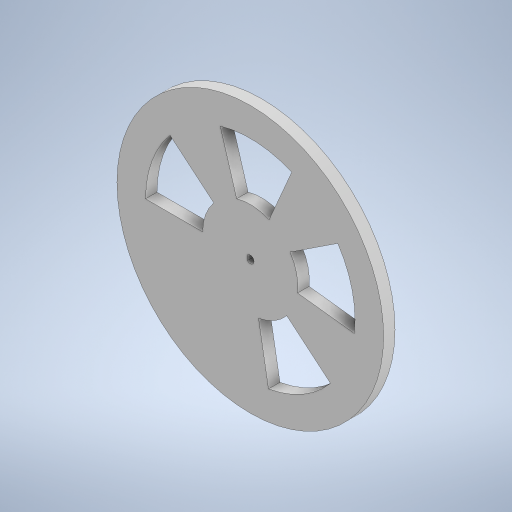
# Autodesk Inventor part: back_cir_hold2
Saved by Autodesk Inventor 2024 (Build 280153000, 153)
## iProperties
Created: 2024-03-23
Part Number: back_cir_hold2
Material: Generic
Document SubType Name: Modeling
Designer: op04o
Density: 1 g/cm^3
Appearance: Default
Author: op04o
Autodesk Inventor part; units mm, degrees
ref_plane "YZ Plane" through (0, 0, 0) normal (1, 0, 0) x (0, 1, 0)
ref_plane "XZ Plane" through (0, 0, 0) normal (0, 1, 0) x (-1, 0, 0)
ref_plane "XY Plane" through (0, 0, 0) normal (0, 0, 1) x (1, 0, 0)
sketch "Sketch1" plane through (0, 0, 0) normal (0, 0, 1) x (1, 0, 0)
  arc A0 (-1.5, -1.3229) -> (-1.5, 1.3229) centre (0, 0) ccw
  line L0 (-1.5, 1.3229) -> (-1.5, -1.3229)
  circle A1 centre (0, 0) radius 70
  dimension "d0" = 4
  dimension "d1" = 1.5
  dimension "d2" = 140
  constraints: 6 coincident, 2 centre point, 2 end point, 2 point on circle, 1 vertical
  measures "d0" diameter of A0
  measures "d1" distance from line of point (0, 0) L0
  measures "d2" diameter of A1
extrude "Extrusion1" add sketch "Sketch1" along normal blind 6
sketch "Sketch2" plane through (0, 0, 0) normal (0, 0, -1) x (-1, 0, 0)
  circle A0 centre (0, 0) radius 70 construction
  arc A1 (1.5, 1.3229) -> (1.5, -1.3229) centre (0, 0) ccw construction
  circle A2 centre (0, 0) radius 70
  line L0 (1.5, -1.3229) -> (1.5, 1.3229) construction
  arc A3 (1.5, 1.3229) -> (1.5, -1.3229) centre (0, 0) ccw construction
  line L1 (0, 0) -> (-1.5321, 1.2856)
  arc A4 (55, 0) -> (42.1324, 35.3533) centre (0, 0) ccw
  line L2 (0, 0) -> (1.5, 0) construction
  line L3 (25, 0) -> (55, 0) construction
  line L4 (0, 0) -> (1.5, 1.2586)
  line L5 (19.1511, 16.0697) -> (42.1324, 35.3533)
  line L6 (0, 0) -> (1.5, 0) construction
  line L7 (25, 0) -> (55, 0) construction
  line L8 (0, 0) -> (1.5, 0)
  line L9 (25, 0) -> (70, 0)
  line L10 (55, 0) -> (25, 0)
  line L11 (-9.902, 22.9554) -> (-21.7844, 50.5019)
  line L12 (15.7742, 52.6894) -> (7.1701, 23.9497)
  arc A5 (15.7742, 52.6894) -> (-21.7844, 50.5019) centre (0, 0) ccw
  line L13 (-24.831, -2.9023) -> (-54.6281, -6.3851)
  line L14 (-45.9518, 30.223) -> (-20.8872, 13.7377)
  arc A6 (-45.9518, 30.223) -> (-54.6281, -6.3851) centre (0, 0) ccw
  line L15 (-4.3412, -24.6202) -> (-9.5506, -54.1644)
  line L16 (-42.1324, -35.3533) -> (-19.1511, -16.0697)
  arc A7 (-42.1324, -35.3533) -> (-9.5506, -54.1644) centre (0, 0) ccw
  arc A8 (-19.1511, -16.0697) -> (-4.3412, -24.6202) centre (0, 0) ccw
  arc A9 (-20.8872, 13.7377) -> (-24.831, -2.9023) centre (0, 0) ccw
  arc A10 (25, 0) -> (19.1511, 16.0697) centre (0, 0) ccw
  arc A11 (7.1701, 23.9497) -> (-9.902, 22.9554) centre (0, 0) ccw
  dimension "d10" = 110
  dimension "d13" = 220
  constraints: 32 end point, 17 point on circle, 9 centre point, 5 collinear, 4 horizontal, 3 coincident, 2 point on line, 1 concentric, 1 midpoint, 25 other
  measures "d10" diameter of A4
extrude "Extrusion4" cut sketch "Sketch2" against normal through all contours L9 A10 L5 A4 | L11 A5 L12 A11 | L13 A6 L14 A9 | L15 A7 L16 A8
body "Solid1"
